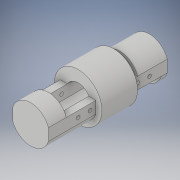
# Autodesk Inventor part: Part2_abbGripp
Saved by Autodesk Inventor 2019 (Build 230136000, 136)
## iProperties
Created: 2019-07-25
Part Number: Part2_abbGripp
Material: Generic
Document SubType Name: Modeling
Designer: romanp
Density: 1 g/cm^3
Appearance: Default
Author: romanp
Autodesk Inventor part; units mm, degrees
ref_plane "YZ Plane" through (0, 0, 0) normal (1, 0, 0) x (0, 1, 0)
ref_plane "XZ Plane" through (0, 0, 0) normal (0, 1, 0) x (-1, 0, 0)
ref_plane "XY Plane" through (0, 0, 0) normal (0, 0, 1) x (1, 0, 0)
ref_plane "Work Plane2" through (0, 0, 20) normal (0, 0, 1) x (1, 0, 0)
sketch "Sketch3" plane through (0, 0, 20) normal (0, 0, 1) x (1, 0, 0)
  line L0 (-11.1369, 5) -> (-11.1369, -5)
  line L1 (-11.1369, 5) -> (-14.9999, 5)
  line L2 (-14.9999, 5) -> (-14.9999, -5)
  line L3 (-14.9999, -5) -> (-11.1369, -5)
  line L4 (-11.1369, -5) -> (-11.1369, 5)
  line L5 (11.1369, 5) -> (14.9999, 5)
  line L6 (14.9999, 5) -> (14.9999, -5)
  line L7 (14.9999, -5) -> (11.1369, -5)
  line L8 (11.1369, -5) -> (11.1369, 5)
  point P0 (0, 0)
  point P1 (0, 0)
  dimension "d9" = 3.863
  dimension "d10" = 3.863
  constraints: 18 end point, 4 parallel, 2 horizontal, 2 perpendicular
  measures "d9" distance of L3.end L2.end
  measures "d10" distance of L6.end L7.end
extrude "Extrusion3" add sketch "Sketch3" against normal blind 30
sketch "Sketch4" plane through (-14.9999, -5, 20) normal (-1, 0, 0) x (0, 0, 1)
  line L0 (0, 5) -> (0, 0)
  circle A0 centre (-15, 5) radius 1.5
  circle A1 centre (-5, 5) radius 1.5
  point P0 (-20, 5)
  dimension "d13" = 5
  dimension "d14" = 5
  dimension "d17" = 3
  dimension "d18" = 3
  constraints: 2 centre point, 2 end point
  measures "d13" distance of L0.end L0.start
  measures "d14" distance of L0.start L0.end
  measures "d17" diameter of A0
  measures "d18" diameter of A1
extrude "Extrusion4" cut sketch "Sketch4" against normal blind 200
sketch "Sketch5" plane through (0, 0, 20) normal (0, 0, 1) x (1, 0, 0)
  circle A0 centre (0, 0) radius 20
  circle A1 centre (0, 0) radius 12.2078
  point P0 (-14.9999, 5)
  point P1 (-11.1369, -5)
  point P2 (11.1369, -5)
  point P3 (14.9999, 5)
  dimension "d21" = 40
  constraints: 2 coincident, 1 centre point, 3 other
  measures "d21" diameter of A0
extrude "Extrusion5" add sketch "Sketch5" along normal blind 30
sketch "Sketch6" plane through (0, 0, 20) normal (0, 0, 1) x (1, 0, 0)
  line L0 (-14.9999, -5) -> (-11.1369, -5) projected
  line L1 (-14.9999, 5) -> (-11.1369, 5) projected
  line L2 (-11.1369, -5) -> (-13.4979, -5)
  line L3 (-13.4979, -5) -> (-13.4979, 5)
  line L4 (-13.4979, 5) -> (-11.1369, 5)
  line L5 (-11.1369, 5) -> (-11.1369, -5)
  line L6 (11.1369, -5) -> (11.1369, 5) projected
  line L7 (11.1369, -5) -> (13.9529, -5)
  line L8 (13.9529, -5) -> (13.9529, 5)
  line L9 (13.9529, 5) -> (11.1369, 5)
  line L10 (11.1369, 5) -> (11.1369, -5)
  arc A0 (11.1369, 5) -> (-11.1369, 5) centre (0, 0) ccw projected
  arc A1 (-11.1369, -5) -> (11.1369, -5) centre (0, 0) ccw projected
  arc A2 (-11.1369, 5) -> (-11.1369, -5) centre (0, 0) ccw
  line L11 (14.9999, -5) -> (11.1369, -5) projected
  line L12 (11.1369, 5) -> (14.9999, 5) projected
  arc A3 (11.1369, -5) -> (11.1369, 5) centre (0, 0) ccw
  constraints: 16 end point, 4 parallel, 4 point on circle, 2 centre point, 2 horizontal, 2 perpendicular, 2 point on line
extrude "Extrusion6" add sketch "Sketch6" along normal blind 30 contours A2 L5 | L6 A3
sketch "Sketch7" plane through (0, 0, 50) normal (0, 0, 1) x (1, 0, 0)
  line L0 (-14.9999, -5) -> (-11.1369, -5) projected
  line L1 (-14.9999, 5) -> (-11.1369, 5) projected
  line L2 (-11.1369, -5) -> (-14.9999, -5)
  line L3 (-14.9999, -5) -> (-14.9999, 5)
  line L4 (-14.9999, 5) -> (-11.1369, 5)
  line L5 (-11.1369, 5) -> (-11.1369, -5)
  arc A0 (-11.1369, -5) -> (11.1369, -5) centre (0, 0) ccw projected
  line L6 (14.9999, 5) -> (14.9999, -5) projected
  line L7 (11.1369, -5) -> (14.9999, -5)
  line L8 (14.9999, -5) -> (14.9999, 5)
  line L9 (14.9999, 5) -> (11.1369, 5)
  line L10 (11.1369, 5) -> (11.1369, -5)
  constraints: 16 end point, 4 parallel, 2 horizontal, 2 perpendicular
extrude "Extrusion7" add sketch "Sketch7" along normal blind 40
sketch "Sketch8" plane through (-14.9999, -5, 50) normal (-1, 0, 0) x (0, 0, 1)
  circle A0 centre (15, 5) radius 1.5
  circle A1 centre (5, 5) radius 1.5
  point P0 (-50, 5)
  point P1 (40, 0)
  dimension "d31" = 3
  dimension "d32" = 3
  constraints: 2 centre point
  measures "d31" diameter of A0
  measures "d32" diameter of A1
extrude "Extrusion8" cut sketch "Sketch8" against normal blind 200
sketch "Sketch10" plane through (0, 0, -10) normal (0, 0, -1) x (-1, 0, 0)
  line L0 (11.1369, -5) -> (11.1369, 5) projected
  line L1 (11.1369, -5) -> (11.9999, -5)
  line L2 (11.9999, -5) -> (11.9999, -3.8424)
  line L3 (11.9999, -3.8424) -> (11.1369, -3.8424)
  line L4 (11.1369, -3.8424) -> (11.1369, -5)
  line L5 (11.9999, -3.8424) -> (11.1369, -3.8424)
  line L6 (11.1369, -3.8424) -> (11.1369, 5)
  line L7 (11.1369, 5) -> (11.9999, 5)
  line L8 (11.9999, 5) -> (11.9999, -3.8424)
  line L9 (-14.9999, -5) -> (-11.1369, -5) projected
  line L10 (-11.1369, 5) -> (-14.9999, 5) projected
  line L11 (-11.1369, -5) -> (-11.9999, -5)
  line L12 (-11.9999, -5) -> (-11.9999, 5)
  line L13 (-11.9999, 5) -> (-11.1369, 5)
  line L14 (-11.1369, 5) -> (-11.1369, -5)
  point P0 (0, 0)
  dimension "d35" = 0.863
  dimension "d36" = 0.863
  constraints: 24 end point, 6 parallel, 3 horizontal, 3 perpendicular, 1 point on line
  measures "d35" distance of L3.end L2.end
  measures "d36" distance of L12.end L13.end
extrude "Extrusion9" cut sketch "Sketch10" against normal blind 200
sketch "Sketch11" plane through (0, 0, 50) normal (0, 0, 1) x (1, 0, 0)
  line L0 (-11.9999, -5) -> (-11.1369, -5) projected
  line L1 (-11.1369, -5) -> (-11.9999, -5)
  line L2 (-11.9999, -5) -> (-11.9999, 5)
  line L3 (-11.9999, 5) -> (-11.1369, 5)
  line L4 (-11.1369, 5) -> (-11.1369, -5)
  line L5 (11.9999, -5) -> (11.1369, -5) projected
  line L6 (11.9999, 5) -> (14.9999, 5) projected
  line L7 (11.1369, -5) -> (11.9999, -5)
  line L8 (11.9999, -5) -> (11.9999, 5)
  line L9 (11.9999, 5) -> (11.1369, 5)
  line L10 (11.1369, 5) -> (11.1369, -5)
  point P0 (0, 0)
  constraints: 16 end point, 4 parallel, 2 horizontal, 2 perpendicular
extrude "Extrusion10" add sketch "Sketch11" against normal blind 30
sketch "Sketch12" plane through (11.9999, -5, -10) normal (-1, 0, 0) x (0, 0, 1)
  line L0 (100, 10) -> (100, 0) projected
  line L1 (0, 10) -> (100, 10)
  line L2 (100, 10) -> (100, 0)
  line L3 (100, 0) -> (0, 0)
  line L4 (0, 0) -> (0, 10)
  circle A0 centre (65, 5) radius 1.5 projected
  circle A1 centre (65, 5) radius 1.5
  circle A2 centre (75, 5) radius 1.5 projected
  circle A3 centre (75, 5) radius 1.5
  circle A4 centre (25, 5) radius 1.5 projected
  circle A5 centre (25, 5) radius 1.5
  circle A6 centre (15, 5) radius 1.5 projected
  circle A7 centre (15, 5) radius 1.5
  point P0 (30, 0)
  constraints: 8 end point, 4 centre point, 4 coincident, 2 parallel, 1 horizontal, 1 perpendicular
extrude "Extrusion11" add sketch "Sketch12" along normal blind 3
sketch "Sketch13" plane through (-11.9999, -5, -10) normal (1, 0, 0) x (0, 0, -1)
  line L0 (-30, 10) -> (0, 10) projected
  line L1 (-100, 0) -> (-100, 10) projected
  line L2 (0, 10) -> (-100, 10)
  line L3 (-100, 10) -> (-100, 0)
  line L4 (-100, 0) -> (0, 0)
  line L5 (0, 0) -> (0, 10)
  circle A0 centre (-65, 5) radius 1.5 projected
  circle A1 centre (-65, 5) radius 1.5
  circle A2 centre (-75, 5) radius 1.5 projected
  circle A3 centre (-75, 5) radius 1.5
  circle A4 centre (-15, 5) radius 1.5 projected
  circle A5 centre (-15, 5) radius 1.5
  circle A6 centre (-25, 5) radius 1.5 projected
  circle A7 centre (-25, 5) radius 1.5
  point P0 (-10, 5)
  constraints: 8 end point, 4 centre point, 4 coincident, 2 parallel, 1 horizontal, 1 perpendicular
extrude "Extrusion12" add sketch "Sketch13" along normal blind 3
sketch "Sketch14" plane through (0, 0, -10) normal (0, 0, -1) x (-1, 0, 0)
  line L0 (14.9999, -5) -> (14.9999, 5) projected
  line L1 (8.9999, -5) -> (8.9999, 5) projected
  line L2 (8.9999, -5) -> (14.9999, -5) projected
  line L3 (14.9999, 5) -> (8.9999, 5) projected
  arc A0 (8.9999, 5) -> (-8.9999, 5) centre (0, 0) ccw
  arc A1 (-8.9999, -5) -> (8.9999, -5) centre (0, 0) ccw
  arc A2 (14.9999, 5) -> (-14.9999, 5) centre (0, 0) ccw
  arc A3 (-14.9999, -5) -> (14.9999, -5) centre (0, 0) ccw
  line L4 (14.9999, 5) -> (8.9999, 5)
  line L5 (-8.9999, 5) -> (-14.9999, 5)
  line L6 (14.9999, -5) -> (8.9999, -5)
  line L7 (-8.9999, -5) -> (-14.9999, -5)
  constraints: 9 end point, 9 point on circle, 4 centre point, 4 collinear, 2 coincident
extrude "Extrusion13" add sketch "Sketch14" against normal blind 5
sketch "Sketch19" plane through (0, 0, -5) normal (0, 0, 1) x (1, 0, 0)
  arc A0 (8.9999, 5) -> (-8.9999, 5) centre (0, 0) ccw
  arc A1 (14.9999, 5) -> (-14.9999, 5) centre (0, 0) ccw
  line L0 (14.9999, 5) -> (8.9999, 5)
  line L1 (-8.9999, 5) -> (-14.9999, 5)
  point P0 (8.9999, 5)
  constraints: 5 point on circle, 4 end point, 2 centre point, 2 coincident, 2 horizontal
extrude "Extrusion17" add sketch "Sketch19" along normal blind 20
sketch "Sketch20" plane through (8.9999, -5, -10) normal (-1, 0, 0) x (0, 0, 1)
  line L0 (100, 10) -> (25, 10) projected
  line L1 (5, 0) -> (100, 0) projected
  line L2 (100, 10) -> (90, 10)
  line L3 (90, 10) -> (90, 0)
  line L4 (90, 0) -> (100, 0)
  line L5 (100, 0) -> (100, 10)
  point P0 (10, 5)
  dimension "d62" = 10
  constraints: 8 end point, 2 parallel, 1 horizontal, 1 perpendicular, 1 point on line
  measures "d62" distance of L4.end L3.end
extrude "Extrusion18" add sketch "Sketch20" along normal blind 20
sketch "Sketch21" plane through (11.1369, -5, 20) normal (0, -1, 0) x (1, 0, 0)
  line L0 (-20.1369, -5) -> (-20.1369, 60) projected
  line L1 (-20.1369, 55) -> (-20.1369, 55)
  line L2 (-15.1369, 60) -> (-15.1369, 60)
  line L3 (-2.137, 60) -> (-20.1369, 60) projected
  line L4 (-2.137, 60) -> (-2.137, -5) projected
  line L5 (-7.137, 60) -> (-7.137, 60)
  line L6 (-2.137, 55) -> (-2.137, 55)
  arc A0 (-15.1369, 60) -> (-20.1369, 55) centre (-15.1369, 55) ccw
  arc A1 (-2.137, 55) -> (-7.137, 60) centre (-7.137, 55) ccw
  line L7 (-20.1369, 55) -> (-20.1369, 60)
  line L8 (-15.1369, 60) -> (-20.1369, 60)
  line L9 (-7.137, 60) -> (-2.137, 60)
  line L10 (-2.137, 60) -> (-2.137, 55)
  point P0 (-11.1369, -20)
  dimension "d65" = 5
  dimension "d66" = 5
  dimension "d67" = 5
  dimension "d68" = 5
  dimension "d69" = 5
  constraints: 16 end point, 8 point on line, 7 tangent, 4 point on circle, 3 collinear, 2 centre point, 1 equal radius, 1 perpendicular
  measures "d65" distance of L0.end L1.end
  measures "d66" distance of L0.end L2.end
  measures "d67" distance of L3.start L5.end
  measures "d68" distance of L3.start L6.end
  measures "d69" radius of A0
extrude "Extrusion19" add sketch "Sketch21" against normal blind 10
sketch "Sketch22" plane through (0, 0, 50) normal (0, 0, 1) x (1, 0, 0)
  arc A0 (14.9999, 5) -> (-14.9999, 5) centre (0, 0) ccw projected
  arc A1 (-14.9999, -5) -> (14.9999, -5) centre (0, 0) ccw
  arc A2 (-8.9999, 5) -> (8.9999, 5) centre (0, 0) ccw
  line L0 (14.9999, 5) -> (-14.9999, 5) projected
  line L1 (-14.9999, 5) -> (14.9999, 5)
  line L2 (-11.1369, -5) -> (-14.9999, -5) projected
  arc A3 (-14.9999, -5) -> (14.9999, -5) centre (0, 0) ccw projected
  line L3 (-14.9999, -5) -> (-8.9999, -5)
  line L4 (8.9999, -5) -> (14.9999, -5)
  constraints: 8 end point, 6 point on circle, 2 centre point, 2 coincident, 2 horizontal, 2 point on line, 1 collinear
extrude "Extrusion20" add sketch "Sketch22" along normal blind 20 contours L4 A1 L2 L3 A2
sketch "Sketch23" plane through (0, 0, 50) normal (0, 0, -1) x (-1, 0, 0)
  arc A0 (-11.1369, -5) -> (11.1369, -5) centre (0, 0) ccw projected
  circle A1 centre (0, 0) radius 12.2078
  line L0 (8.9999, 5) -> (8.9999, -5) projected
  circle A2 centre (0, 0) radius 10.2956
  line L1 (8.9999, -5) -> (11.1369, -5) projected
  line L2 (-11.1369, 5) -> (-14.9999, 5) projected
  arc A3 (11.1369, 5) -> (-11.1369, 5) centre (0, 0) ccw projected
  line L3 (11.1369, -5) -> (8.9999, -5)
  line L4 (-8.9999, -5) -> (-11.1369, -5)
  line L5 (-11.1369, 5) -> (-8.9999, 5)
  line L6 (8.9999, 5) -> (11.1369, 5)
  constraints: 8 end point, 5 point on circle, 4 horizontal, 2 centre point, 2 coincident
extrude "Extrusion21" add sketch "Sketch23" along normal blind 30 contours L4 A2 L1 A0 | A1 L6 A2 L5
sketch "Sketch24" plane through (-14.9999, 5, 90) normal (0, 1, 0) x (1, 0, 0)
  point P0 (14.9999, 90)
sketch "Sketch25" plane through (0, 0, 90) normal (0, 0, 1) x (1, 0, 0)
  arc A0 (-14.9999, -5) -> (14.9999, -5) centre (0, 0) ccw projected
  line L0 (-8.9999, 5) -> (-8.9999, -5) projected
  line L1 (14.9999, 5) -> (-14.9999, 5) projected
  line L2 (14.9999, 5) -> (-14.9999, 5)
  line L3 (-14.9999, -5) -> (-8.9999, -5) projected
  line L4 (14.9999, -5) -> (-14.9999, -5)
  arc A1 (-14.9999, -5) -> (14.9999, -5) centre (0, 0) ccw
  arc A2 (14.9999, 5) -> (-14.9999, 5) centre (0, 0) ccw
  constraints: 5 end point, 4 point on circle, 2 centre point, 2 collinear, 1 coincident
extrude "Extrusion22" add sketch "Sketch25" against normal blind 15
sketch "Sketch26" plane through (8.9999, 5, 50) normal (0, 1, 0) x (1, 0, 0)
  arc A0 (-5, -30) -> (0, -25) centre (-5, -25) ccw projected
  line L0 (0, -25) -> (-17.9999, -25)
  line L1 (-12.9999, -30) -> (-5, -30)
  arc A1 (-5, -30) -> (0, -25) centre (-5, -25) ccw
  line L2 (-23.9999, -25) -> (-17.9999, -25) projected
  arc A2 (-17.9999, -25) -> (-12.9999, -30) centre (-12.9999, -25) ccw
  line L3 (-5, -30) -> (-12.9999, -30)
  point P0 (-8.9999, 50)
  constraints: 6 end point, 6 point on circle, 2 centre point, 2 horizontal, 1 concentric, 1 parallel, 1 other
extrude "Extrusion23" add sketch "Sketch26" against normal blind 10
sketch "Sketch28" plane through (0, 0, 70) normal (0, 0, 1) x (1, 0, 0)
  line L0 (-14.8626, -5) -> (-8.9999, -5)
  line L1 (8.9999, -5) -> (14.9999, -5) projected
  line L2 (8.9999, -5) -> (14.9999, -5)
  arc A0 (-14.9999, -5) -> (14.9999, -5) centre (0, 0) ccw
  line L3 (-14.9999, -5) -> (-8.9999, -5) projected
  line L4 (-14.8626, -5) -> (-14.9999, -5)
  arc A1 (-8.9999, -5) -> (8.9999, -5) centre (0, 0) ccw
  point P0 (0, 0)
  constraints: 6 end point, 4 point on circle, 2 centre point, 2 horizontal, 1 collinear
extrude "Extrusion24" add sketch "Sketch28" along normal blind 5
body "Solid1"
